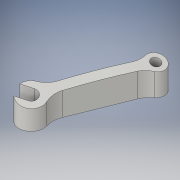
# Autodesk Inventor part: Team Pin Mechanical-Left Wrench
Saved by Autodesk Inventor 2016 (Build 200138000, 138)
## iProperties
Created: 2016-02-20
Part Number: Team Pin Mechanical-Left Wrench
Material: Generic
Document SubType Name: Modeling
Designer: RoksBot
Density: 1 g/cm^3
Appearance: White
Author: RoksBot
Autodesk Inventor part; units mm, degrees
ref_plane "YZ Plane" through (0, 0, 0) normal (1, 0, 0) x (0, 1, 0)
ref_plane "XZ Plane" through (0, 0, 0) normal (0, 1, 0) x (-1, 0, 0)
ref_plane "XY Plane" through (0, 0, 0) normal (0, 0, 1) x (1, 0, 0)
sketch "Sketch1" plane through (0, 0, 0) normal (0, 0, 1) x (1, 0, 0)
  line L0 (0, 0) -> (0, 8.6646) construction
  line L1 (20.9931, 1.27) -> (20.9931, 5.715)
  line L2 (20.9931, 5.715) -> (27.9781, 3.81)
  line L3 (27.9781, 3.81) -> (27.9781, 0)
  line L4 (27.9781, 0) -> (20.9931, 0)
  line L5 (20.9931, 1.27) -> (18.4531, 1.27)
  line L6 (18.4531, 1.27) -> (18.4531, 0)
  line L7 (18.4531, 0) -> (20.9931, 0)
  dimension "d0" = 20.9931
  dimension "d1" = 4.445
  dimension "d2" = 1.27
  dimension "d3" = 2.54
  dimension "d4" = 3.81
  dimension "d5" = 6.985
  constraints: 16 end point, 2 parallel, 2 perpendicular, 2 vertical, 1 horizontal, 1 horizontal alignment
  measures "d0" distance between parallel lines of L0 L1
  measures "d1" distance from line of L5 L1.end
  measures "d2" distance of L5.end L6.end
  measures "d3" distance between parallel lines of L1 L6
  measures "d4" distance of L2.end L3.end
  measures "d5" distance between parallel lines of L1 L3
revolve "Revolution1" add sketch "Sketch1" angle 360 about axis through (0, 0, 0) along (0, 1, 0)
ref_plane "Work Plane1" through (0, 3.81, 0) normal (0, 1, 0) x (1, 0, 0)
sketch "Sketch2" plane through (0, 0, 0) normal (0, -1, 0) x (1, 0, 0)
  line L0 (0, 0) -> (-45.8206, 0) construction
  circle A0 centre (0, 0) radius 27.9781 projected
  line L1 (-27.6227, 4.445) -> (-30.5181, 2.54)
  line L2 (-30.5181, 2.54) -> (-30.5181, -2.54)
  line L3 (-30.5181, -2.54) -> (-27.6227, -4.445)
  dimension "d7" = 2.54
  dimension "d8" = 8.89
  dimension "d9" = 5.08
  constraints: 8 end point, 2 point on circle, 1 equal length, 1 horizontal, 1 vertical, 1 other
  measures "d7" distance edge to line of A0 L2
  measures "d8" distance of L3.end L1.start
  measures "d9" distance of L1.end L2.end
extrude "Extrusion1" add sketch "Sketch2" against normal up to surface (3.81 mm away) contours A0 L3 L2 L1
pattern_circular "Circular Pattern1" count 12 over 360 about axis through (0, 1.905, 0) along (0, -1, 0) of "Extrusion1"
sketch "Sketch3" plane through (0, 1.27, 0) normal (0, 1, 0) x (1, 0, 0)
  circle A0 centre (0, 0) radius 18.4531 projected
  circle A1 centre (0, 0) radius 18.4531 projected
  circle A2 centre (0, 0) radius 20.9931 projected
  circle A3 centre (0, 0) radius 20.9931 projected
  arc A4 (-26.1445, 9.9619) -> (-27.6227, 4.445) centre (0, 0) ccw projected
  arc A5 (-27.6227, 4.445) -> (-27.6227, -4.445) centre (0, 0) ccw projected
  arc A6 (-27.6227, -4.445) -> (-26.1445, -9.9619) centre (0, 0) ccw projected
  arc A7 (-26.1445, -9.9619) -> (-21.6995, -17.6609) centre (0, 0) ccw projected
  arc A8 (-21.6995, -17.6609) -> (-17.6609, -21.6995) centre (0, 0) ccw projected
  arc A9 (-17.6609, -21.6995) -> (-9.9619, -26.1445) centre (0, 0) ccw projected
  arc A10 (-9.9619, -26.1445) -> (-4.445, -27.6227) centre (0, 0) ccw projected
  arc A11 (-4.445, -27.6227) -> (4.445, -27.6227) centre (0, 0) ccw projected
  arc A12 (4.445, -27.6227) -> (9.9619, -26.1445) centre (0, 0) ccw projected
  arc A13 (9.9619, -26.1445) -> (17.6609, -21.6995) centre (0, 0) ccw projected
  arc A14 (17.6609, -21.6995) -> (21.6995, -17.6609) centre (0, 0) ccw projected
  arc A15 (21.6995, -17.6609) -> (26.1445, -9.9619) centre (0, 0) ccw projected
  arc A16 (26.1445, -9.9619) -> (27.6227, -4.445) centre (0, 0) ccw projected
  arc A17 (27.6227, -4.445) -> (27.6227, 4.445) centre (0, 0) ccw projected
  arc A18 (27.6227, 4.445) -> (26.1445, 9.9619) centre (0, 0) ccw projected
  arc A19 (26.1445, 9.9619) -> (21.6995, 17.6609) centre (0, 0) ccw projected
  arc A20 (21.6995, 17.6609) -> (17.6609, 21.6995) centre (0, 0) ccw projected
  arc A21 (17.6609, 21.6995) -> (9.9619, 26.1445) centre (0, 0) ccw projected
  arc A22 (9.9619, 26.1445) -> (4.445, 27.6227) centre (0, 0) ccw projected
  arc A23 (4.445, 27.6227) -> (-4.445, 27.6227) centre (0, 0) ccw projected
  arc A24 (-4.445, 27.6227) -> (-9.9619, 26.1445) centre (0, 0) ccw projected
  arc A25 (-9.9619, 26.1445) -> (-17.6609, 21.6995) centre (0, 0) ccw projected
  arc A26 (-17.6609, 21.6995) -> (-21.6995, 17.6609) centre (0, 0) ccw projected
  arc A27 (-21.6995, 17.6609) -> (-26.1445, 9.9619) centre (0, 0) ccw projected
  circle A28 centre (0, 0) radius 22.8981
  spline S0 degree 2 poles (-20.4865, -10.8927) (-20.2314, -10.7347) (-20.0767, -10.9844) knots 0 0 0 1 1 1
  spline S1 degree 2 poles (-20.0767, -10.9844) (-19.9219, -11.2342) (-20.177, -11.3922) knots 0 0 0 1 1 1
  line L0 (-20.177, -11.3922) -> (-22.4984, -12.8306)
  line L1 (-22.4984, -12.8306) -> (-21.0657, -12.8234)
  spline S2 degree 2 poles (-21.0657, -12.8234) (-20.8353, -12.8371) (-20.7343, -13.0001) knots 0 0 0 1 1 1
  spline S3 degree 2 poles (-20.7343, -13.0001) (-20.6366, -13.1578) (-20.7235, -13.3463) knots 0 0 0 1 1 1
  line L2 (-20.7235, -13.3463) -> (-21.4078, -14.6436)
  line L3 (-21.4078, -14.6436) -> (-19.0627, -13.1905)
  spline S4 degree 2 poles (-19.0627, -13.1905) (-18.8077, -13.0325) (-18.6529, -13.2822) knots 0 0 0 1 1 1
  spline S5 degree 2 poles (-18.6529, -13.2822) (-18.4949, -13.5373) (-18.7499, -13.6953) knots 0 0 0 1 1 1
  line L4 (-18.7499, -13.6953) -> (-21.6577, -15.497)
  spline S6 degree 2 poles (-21.6577, -15.497) (-21.9259, -15.6631) (-22.0936, -15.3923) knots 0 0 0 1 1 1
  spline S7 degree 2 poles (-22.0936, -15.3923) (-22.2093, -15.2057) (-22.1246, -15.0076) knots 0 0 0 1 1 1
  line L5 (-22.1246, -15.0076) -> (-21.3965, -13.3994)
  line L6 (-21.3965, -13.3994) -> (-23.1279, -13.3298)
  spline S8 degree 2 poles (-23.1279, -13.3298) (-23.414, -13.3142) (-23.5248, -13.1355) knots 0 0 0 1 1 1
  spline S9 degree 2 poles (-23.5248, -13.1355) (-23.5932, -13.025) (-23.5178, -12.7709) (-23.3942, -12.6944) knots 0 0 0 1 2 2 2
  line L7 (-23.3942, -12.6944) -> (-20.4865, -10.8927)
  line L8 (-21.4115, -8.1592) -> (-20.6563, -9.942)
  line L9 (-20.6563, -9.942) -> (-23.6894, -11.2268)
  line L10 (-23.6894, -11.2268) -> (-24.4445, -9.444)
  spline S10 degree 2 poles (-24.4445, -9.444) (-24.5591, -9.1734) (-24.2914, -9.06) knots 0 0 0 1 1 1
  spline S11 degree 2 poles (-24.2914, -9.06) (-24.0209, -8.9454) (-23.9063, -9.216) knots 0 0 0 1 1 1
  line L11 (-23.9063, -9.216) -> (-23.3743, -10.4719)
  line L12 (-23.3743, -10.4719) -> (-22.8189, -10.2367)
  line L13 (-22.8189, -10.2367) -> (-23.3171, -9.0605)
  spline S12 degree 2 poles (-23.3171, -9.0605) (-23.4293, -8.7956) (-23.1616, -8.6822) knots 0 0 0 1 1 1
  spline S13 degree 2 poles (-23.1616, -8.6822) (-22.8854, -8.5652) (-22.7732, -8.8301) knots 0 0 0 1 1 1
  line L14 (-22.7732, -8.8301) -> (-22.275, -10.0063)
  line L15 (-22.275, -10.0063) -> (-21.4235, -9.6456)
  line L16 (-21.4235, -9.6456) -> (-21.9554, -8.3897)
  spline S14 degree 2 poles (-21.9554, -8.3897) (-22.07, -8.1191) (-21.8023, -8.0057) knots 0 0 0 1 1 1
  spline S15 degree 2 poles (-21.8023, -8.0057) (-21.5261, -7.8887) (-21.4115, -8.1592) knots 0 0 0 1 1 1
  spline S16 degree 2 poles (-22.8056, -5.2377) (-22.4484, -5.3877) (-22.1014, -5.7752) (-22.015, -6.0818) knots 0 0 0 1 2 2 2
  spline S17 degree 2 poles (-22.015, -6.0818) (-21.8732, -6.5849) (-22.313, -7.0655) knots 0 0 0 1 1 1
  spline S18 degree 2 poles (-22.313, -7.0655) (-22.5945, -7.4918) (-23.3387, -7.7016) knots 0 0 0 1 1 1
  spline S19 degree 2 poles (-23.3387, -7.7016) (-24.1544, -7.9314) (-24.69, -7.6614) knots 0 0 0 1 1 1
  spline S20 degree 2 poles (-24.69, -7.6614) (-25.1213, -7.4423) (-25.2479, -6.9928) knots 0 0 0 1 1 1
  spline S21 degree 2 poles (-25.2479, -6.9928) (-25.3444, -6.6505) (-25.2198, -6.1462) (-24.9563, -5.8953) knots 0 0 0 1 2 2 2
  spline S22 degree 2 poles (-24.9563, -5.8953) (-24.9018, -5.8381) (-24.8303, -5.818) knots 0 0 0 1 1 1
  spline S23 degree 2 poles (-24.8303, -5.818) (-24.7112, -5.7844) (-24.4997, -5.908) (-24.4678, -6.0211) knots 0 0 0 1 2 2 2
  spline S24 degree 2 poles (-24.4678, -6.0211) (-24.4242, -6.1759) (-24.5806, -6.3164) knots 0 0 0 1 1 1
  spline S25 degree 2 poles (-24.5806, -6.3164) (-24.7683, -6.517) (-24.6827, -6.8207) knots 0 0 0 1 1 1
  spline S26 degree 2 poles (-24.6827, -6.8207) (-24.6139, -7.0648) (-24.3475, -7.1664) knots 0 0 0 1 1 1
  spline S27 degree 2 poles (-24.3475, -7.1664) (-24.0157, -7.2947) (-23.4948, -7.1479) knots 0 0 0 1 1 1
  spline S28 degree 2 poles (-23.4948, -7.1479) (-23.0095, -7.0111) (-22.5148, -6.4861) (-22.587, -6.2301) knots 0 0 0 1 2 2 2
  spline S29 degree 2 poles (-22.587, -6.2301) (-22.6767, -5.9116) (-22.9983, -5.774) knots 0 0 0 1 1 1
  spline S30 degree 2 poles (-22.9983, -5.774) (-23.1807, -5.7194) (-23.2168, -5.5914) knots 0 0 0 1 1 1
  spline S31 degree 2 poles (-23.2168, -5.5914) (-23.2487, -5.4783) (-23.1196, -5.2523) (-23.0064, -5.2204) knots 0 0 0 1 2 2 2
  spline S32 degree 2 poles (-23.0064, -5.2204) (-22.9082, -5.1928) (-22.8056, -5.2377) knots 0 0 0 1 1 1
  spline S33 degree 2 poles (-23.0841, -2.194) (-22.7873, -2.1504) (-22.7455, -2.435) knots 0 0 0 1 1 1
  spline S34 degree 2 poles (-22.7455, -2.435) (-22.7028, -2.7257) (-22.9996, -2.7693) knots 0 0 0 1 1 1
  line L17 (-22.9996, -2.7693) -> (-24.1563, -2.9392)
  line L18 (-24.1563, -2.9392) -> (-23.9877, -4.0867)
  line L19 (-23.9877, -4.0867) -> (-22.8311, -3.9168)
  spline S35 degree 2 poles (-22.8311, -3.9168) (-22.5342, -3.8732) (-22.4915, -4.1639) knots 0 0 0 1 1 1
  spline S36 degree 2 poles (-22.4915, -4.1639) (-22.4488, -4.4546) (-22.7456, -4.4982) knots 0 0 0 1 1 1
  line L20 (-22.7456, -4.4982) -> (-25.4599, -4.8969)
  spline S37 degree 2 poles (-25.4599, -4.8969) (-25.7536, -4.9401) (-25.7963, -4.6494) knots 0 0 0 1 1 1
  spline S38 degree 2 poles (-25.7963, -4.6494) (-25.839, -4.3587) (-25.5453, -4.3155) knots 0 0 0 1 1 1
  line L21 (-25.5453, -4.3155) -> (-24.5722, -4.1726)
  line L22 (-24.5722, -4.1726) -> (-24.7408, -3.0251)
  line L23 (-24.7408, -3.0251) -> (-25.7139, -3.168)
  spline S39 degree 2 poles (-25.7139, -3.168) (-26.0076, -3.2112) (-26.0503, -2.9205) knots 0 0 0 1 1 1
  spline S40 degree 2 poles (-26.0503, -2.9205) (-26.0921, -2.6359) (-25.7984, -2.5928) knots 0 0 0 1 1 1
  line L24 (-25.7984, -2.5928) -> (-23.0841, -2.194)
  spline S41 degree 2 poles (-23.2836, 1.208) (-23.2064, 1.2364) (-23.1539, 1.2367) knots 0 0 0 1 1 1
  spline S42 degree 2 poles (-23.1539, 1.2367) (-23.0302, 1.2375) (-22.8651, 1.053) (-22.8643, 0.9323) knots 0 0 0 1 2 2 2
  spline S43 degree 2 poles (-22.8643, 0.9323) (-22.8631, 0.7437) (-23.042, 0.6683) knots 0 0 0 1 1 1
  line L25 (-23.042, 0.6683) -> (-23.4523, 0.5049)
  line L26 (-23.4523, 0.5049) -> (-23.4439, -0.8127)
  line L27 (-23.4439, -0.8127) -> (-23.0192, -0.9677)
  spline S44 degree 2 poles (-23.0192, -0.9677) (-22.8518, -1.0347) (-22.8505, -1.2295) knots 0 0 0 1 1 1
  spline S45 degree 2 poles (-22.8505, -1.2295) (-22.8498, -1.3439) (-23.0064, -1.5305) (-23.1301, -1.5313) knots 0 0 0 1 2 2 2
  spline S46 degree 2 poles (-23.1301, -1.5313) (-23.1826, -1.5316) (-23.2322, -1.5134) knots 0 0 0 1 1 1
  line L28 (-23.2322, -1.5134) -> (-26.0565, -0.4767)
  spline S47 degree 2 poles (-26.0565, -0.4767) (-26.2212, -0.3571) (-26.2222, -0.1963) knots 0 0 0 1 1 1
  spline S48 degree 2 poles (-26.2222, -0.1963) (-26.2233, -0.0262) (-26.0632, 0.0924) knots 0 0 0 1 1 1
  line L29 (-26.0632, 0.0924) -> (-23.2836, 1.208)
  line L30 (-24.0233, 0.3126) -> (-25.2852, -0.1749)
  line L31 (-25.2852, -0.1749) -> (-24.0173, -0.6307)
  line L32 (-24.0173, -0.6307) -> (-24.0233, 0.3126)
  spline S49 degree 2 poles (-22.7917, 4.2665) (-22.4883, 4.2255) (-22.5223, 3.9742) knots 0 0 0 1 1 1
  spline S50 degree 2 poles (-22.5223, 3.9742) (-22.5451, 3.8056) (-22.7963, 3.7022) knots 0 0 0 1 1 1
  line L33 (-22.7963, 3.7022) -> (-24.9996, 2.6644)
  line L34 (-24.9996, 2.6644) -> (-23.038, 2.3991)
  spline S51 degree 2 poles (-23.038, 2.3991) (-22.7407, 2.3589) (-22.7793, 2.0739) knots 0 0 0 1 1 1
  spline S52 degree 2 poles (-22.7793, 2.0739) (-22.8178, 1.7888) (-23.1151, 1.8291) knots 0 0 0 1 1 1
  line L35 (-23.1151, 1.8291) -> (-25.8582, 2.2)
  spline S53 degree 2 poles (-25.8582, 2.2) (-26.1463, 2.239) (-26.109, 2.5148) knots 0 0 0 1 1 1
  spline S54 degree 2 poles (-26.109, 2.5148) (-26.0867, 2.6803) (-25.9475, 2.6709) knots 0 0 0 1 1 1
  line L36 (-25.9475, 2.6709) -> (-23.6718, 3.805)
  line L37 (-23.6718, 3.805) -> (-25.5813, 4.0632)
  spline S55 degree 2 poles (-25.5813, 4.0632) (-25.8755, 4.103) (-25.837, 4.3881) knots 0 0 0 1 1 1
  spline S56 degree 2 poles (-25.837, 4.3881) (-25.7984, 4.6731) (-25.5042, 4.6333) knots 0 0 0 1 1 1
  line L38 (-25.5042, 4.6333) -> (-22.7917, 4.2665)
  spline S57 degree 2 poles (-22.4654, 5.6266) (-22.1736, 5.5569) (-22.2419, 5.2711) knots 0 0 0 1 1 1
  spline S58 degree 2 poles (-22.2419, 5.2711) (-22.3101, 4.9853) (-22.6019, 5.055) knots 0 0 0 1 1 1
  line L39 (-22.6019, 5.055) -> (-25.2702, 5.6925)
  spline S59 degree 2 poles (-25.2702, 5.6925) (-25.559, 5.7615) (-25.4907, 6.0473) knots 0 0 0 1 1 1
  spline S60 degree 2 poles (-25.4907, 6.0473) (-25.4224, 6.3331) (-25.1336, 6.2641) knots 0 0 0 1 1 1
  line L40 (-25.1336, 6.2641) -> (-22.4654, 5.6266)
  spline S61 degree 2 poles (-21.7348, 8.6674) (-21.5264, 8.3409) (-21.4615, 7.8248) (-21.5649, 7.5235) knots 0 0 0 1 2 2 2
  spline S62 degree 2 poles (-21.5649, 7.5235) (-21.7346, 7.0291) (-22.3696, 6.8841) knots 0 0 0 1 1 1
  spline S63 degree 2 poles (-22.3696, 6.8841) (-22.8437, 6.6936) (-23.5751, 6.9445) knots 0 0 0 1 1 1
  spline S64 degree 2 poles (-23.5751, 6.9445) (-24.3766, 7.2196) (-24.6635, 7.7463) knots 0 0 0 1 1 1
  spline S65 degree 2 poles (-24.6635, 7.7463) (-24.8935, 8.1719) (-24.7419, 8.6136) knots 0 0 0 1 1 1
  spline S66 degree 2 poles (-24.7419, 8.6136) (-24.6265, 8.95) (-24.2371, 9.2938) (-23.8777, 9.3503) knots 0 0 0 1 2 2 2
  spline S67 degree 2 poles (-23.8777, 9.3503) (-23.8003, 9.3663) (-23.7301, 9.3422) knots 0 0 0 1 1 1
  spline S68 degree 2 poles (-23.7301, 9.3422) (-23.6131, 9.3021) (-23.5094, 9.0801) (-23.5475, 8.9689) knots 0 0 0 1 2 2 2
  spline S69 degree 2 poles (-23.5475, 8.9689) (-23.5997, 8.8168) (-23.8083, 8.7903) knots 0 0 0 1 1 1
  spline S70 degree 2 poles (-23.8083, 8.7903) (-24.0768, 8.732) (-24.1792, 8.4336) knots 0 0 0 1 1 1
  spline S71 degree 2 poles (-24.1792, 8.4336) (-24.2615, 8.1937) (-24.1002, 7.9585) knots 0 0 0 1 1 1
  spline S72 degree 2 poles (-24.1002, 7.9585) (-23.9003, 7.6643) (-23.3884, 7.4887) knots 0 0 0 1 1 1
  spline S73 degree 2 poles (-23.3884, 7.4887) (-22.9115, 7.3251) (-22.206, 7.4754) (-22.1197, 7.7269) knots 0 0 0 1 2 2 2
  spline S74 degree 2 poles (-22.1197, 7.7269) (-22.0123, 8.04) (-22.1984, 8.336) knots 0 0 0 1 1 1
  spline S75 degree 2 poles (-22.1984, 8.336) (-22.3174, 8.4847) (-22.2743, 8.6105) knots 0 0 0 1 1 1
  spline S76 degree 2 poles (-22.2743, 8.6105) (-22.2361, 8.7217) (-22.0014, 8.8341) (-21.8902, 8.7959) knots 0 0 0 1 2 2 2
  spline S77 degree 2 poles (-21.8902, 8.7959) (-21.7937, 8.7628) (-21.7348, 8.6674) knots 0 0 0 1 1 1
  spline S78 degree 2 poles (-20.1702, 11.694) (-20.0886, 11.684) (-20.0417, 11.6603) knots 0 0 0 1 1 1
  spline S79 degree 2 poles (-20.0417, 11.6603) (-19.9312, 11.6046) (-19.8684, 11.3651) (-19.9228, 11.2574) knots 0 0 0 1 2 2 2
  spline S80 degree 2 poles (-19.9228, 11.2574) (-20.0077, 11.0889) (-20.2013, 11.1035) knots 0 0 0 1 1 1
  line L41 (-20.2013, 11.1035) -> (-20.641, 11.1451)
  line L42 (-20.641, 11.1451) -> (-21.2344, 9.9688)
  line L43 (-21.2344, 9.9688) -> (-20.9272, 9.6371)
  spline S81 degree 2 poles (-20.9272, 9.6371) (-20.8087, 9.5011) (-20.8965, 9.3272) knots 0 0 0 1 1 1
  spline S82 degree 2 poles (-20.8965, 9.3272) (-20.948, 9.225) (-21.1724, 9.1304) (-21.2829, 9.1861) knots 0 0 0 1 2 2 2
  spline S83 degree 2 poles (-21.2829, 9.1861) (-21.3298, 9.2098) (-21.3656, 9.2486) knots 0 0 0 1 1 1
  line L44 (-21.3656, 9.2486) -> (-23.4063, 11.4593)
  spline S84 degree 2 poles (-23.4063, 11.4593) (-23.4983, 11.6408) (-23.4258, 11.7844) knots 0 0 0 1 1 1
  spline S85 degree 2 poles (-23.4258, 11.7844) (-23.3492, 11.9363) (-23.1527, 11.9688) knots 0 0 0 1 1 1
  line L45 (-23.1527, 11.9688) -> (-20.1702, 11.694)
  line L46 (-21.2369, 11.2344) -> (-22.5822, 11.3761)
  line L47 (-22.5822, 11.3761) -> (-21.6617, 10.3922)
  line L48 (-21.6617, 10.3922) -> (-21.2369, 11.2344)
  line L49 (-18.3775, 13.6927) -> (-19.469, 12.0936)
  line L50 (-19.469, 12.0936) -> (-21.9443, 13.7831)
  spline S86 degree 2 poles (-21.9443, 13.7831) (-22.1896, 13.9505) (-22.0274, 14.188) knots 0 0 0 1 1 1
  spline S87 degree 2 poles (-22.0274, 14.188) (-21.867, 14.4231) (-21.6218, 14.2557) knots 0 0 0 1 1 1
  line L51 (-21.6218, 14.2557) -> (-19.6343, 12.8992)
  line L52 (-19.6343, 12.8992) -> (-18.8654, 14.0258)
  spline S88 degree 2 poles (-18.8654, 14.0258) (-18.6998, 14.2684) (-18.4597, 14.1045) knots 0 0 0 1 1 1
  spline S89 degree 2 poles (-18.4597, 14.1045) (-18.2119, 13.9354) (-18.3775, 13.6927) knots 0 0 0 1 1 1
  dimension "d16" = 1.905
  constraints: 1 centre point, 1 coincident, 1 other
  measures "d16" radial gap between concentric circles of A2 A28
extrude "Extrusion2" cut sketch "Sketch3" along normal blind 25.4 contours S5 L4 S6 S7 L5 L6 S8 S9 L7 S0 A28 S1 L0 L1 S2 S3 L2 L3 S4 | L8 L9 L10 S10 S11 L11 L12 L13 S12 S13 L14 L15 L16 S14 S15 | L49 L50 S86 S87 L51 L52 S88 S89 | A28 S0 S1 | S79 S80 A28 | A28 S80 L41 L42 L43 S81 S82 S83 L44 S84 S85 L45 S78 S79 | S17 S18 S19 S20 S21 S22 S23 S24 S25 S26 S27 S28 S29 S30 S31 S32 S16 A28 | A28 S16 S17 | S81 S82 A28 | S36 L20 S37 S38 L21 L22 L23 S39 S40 L24 S33 A28 S34 L17 L18 L19 S35 | A28 S35 S36 | S61 S62 A28 | A28 S62 S63 S64 S65 S66 S67 S68 S69 S70 S71 S72 S73 S74 S75 S76 S77 S61 | A28 S33 S34 | S57 S58 A28 | A28 S58 L39 S59 S60 L40 S57 | S45 S46 L28 S47 S48 L29 S41 S42 A28 S43 L25 L26 L27 S44 | A28 S44 S45 | S49 S50 A28 | A28 S50 L33 L34 S51 S52 L35 S53 S54 L36 L37 S55 S56 L38 S49 | A28 S42 S43 | S51 S52 A28
sketch "Sketch4" plane through (0, 1.27, 0) normal (0, 1, 0) x (1, 0, 0)
  line L0 (-22.7963, 3.7022) -> (-24.9996, 2.6644) projected
  line L1 (-24.9996, 2.6644) -> (-23.038, 2.3991) projected
  line L2 (-23.1151, 1.8291) -> (-25.8582, 2.2) projected
  line L3 (-25.9475, 2.6709) -> (-23.6718, 3.805) projected
  line L4 (-23.6718, 3.805) -> (-25.5813, 4.0632) projected
  line L5 (-25.5042, 4.6333) -> (-22.7917, 4.2665) projected
  line L6 (-23.042, 0.6683) -> (-23.4523, 0.5049) projected
  line L7 (-23.4523, 0.5049) -> (-23.4439, -0.8127) projected
  line L8 (-23.4439, -0.8127) -> (-23.0192, -0.9677) projected
  line L9 (-23.2322, -1.5134) -> (-26.0565, -0.4767) projected
  line L10 (-26.0632, 0.0924) -> (-23.2836, 1.208) projected
  line L11 (-20.177, -11.3922) -> (-22.4984, -12.8306) projected
  line L12 (-22.4984, -12.8306) -> (-21.0657, -12.8234) projected
  line L13 (-20.7235, -13.3463) -> (-21.4078, -14.6436) projected
  line L14 (-21.4078, -14.6436) -> (-19.0627, -13.1905) projected
  line L15 (-18.7499, -13.6953) -> (-21.6577, -15.497) projected
  line L16 (-22.1246, -15.0076) -> (-21.3965, -13.3994) projected
  line L17 (-21.3965, -13.3994) -> (-23.1279, -13.3298) projected
  line L18 (-23.3942, -12.6944) -> (-20.4865, -10.8927) projected
  line L19 (-20.6563, -9.942) -> (-23.6894, -11.2268) projected
  line L20 (-23.6894, -11.2268) -> (-24.4445, -9.444) projected
  line L21 (-23.9063, -9.216) -> (-23.3743, -10.4719) projected
  line L22 (-23.3743, -10.4719) -> (-22.8189, -10.2367) projected
  line L23 (-22.8189, -10.2367) -> (-23.3171, -9.0605) projected
  line L24 (-22.7732, -8.8301) -> (-22.275, -10.0063) projected
  line L25 (-22.275, -10.0063) -> (-21.4235, -9.6456) projected
  line L26 (-21.4235, -9.6456) -> (-21.9554, -8.3897) projected
  line L27 (-21.4115, -8.1592) -> (-20.6563, -9.942) projected
  line L28 (-22.9996, -2.7693) -> (-24.1563, -2.9392) projected
  line L29 (-24.1563, -2.9392) -> (-23.9877, -4.0867) projected
  line L30 (-23.9877, -4.0867) -> (-22.8311, -3.9168) projected
  line L31 (-22.7456, -4.4982) -> (-25.4599, -4.8969) projected
  line L32 (-25.5453, -4.3155) -> (-24.5722, -4.1726) projected
  line L33 (-24.5722, -4.1726) -> (-24.7408, -3.0251) projected
  line L34 (-24.7408, -3.0251) -> (-25.7139, -3.168) projected
  line L35 (-25.7984, -2.5928) -> (-23.0841, -2.194) projected
  line L36 (-22.6019, 5.055) -> (-25.2702, 5.6925) projected
  line L37 (-25.1336, 6.2641) -> (-22.4654, 5.6266) projected
  line L38 (-20.2013, 11.1035) -> (-20.641, 11.1451) projected
  line L39 (-20.641, 11.1451) -> (-21.2344, 9.9688) projected
  line L40 (-21.2344, 9.9688) -> (-20.9272, 9.6371) projected
  line L41 (-21.3656, 9.2486) -> (-23.4063, 11.4593) projected
  line L42 (-23.1527, 11.9688) -> (-20.1702, 11.694) projected
  line L43 (-19.469, 12.0936) -> (-21.9443, 13.7831) projected
  line L44 (-21.6218, 14.2557) -> (-19.6343, 12.8992) projected
  line L45 (-19.6343, 12.8992) -> (-18.8654, 14.0258) projected
  line L46 (-18.3775, 13.6927) -> (-19.469, 12.0936) projected
  circle A0 centre (0, 0) radius 20.9931 projected
  arc A1 (-26.1445, 9.9619) -> (-27.6227, 4.445) centre (0, 0) ccw projected
  arc A2 (-27.6227, 4.445) -> (-27.6227, -4.445) centre (0, 0) ccw projected
  arc A3 (-27.6227, -4.445) -> (-26.1445, -9.9619) centre (0, 0) ccw projected
  arc A4 (-26.1445, -9.9619) -> (-21.6995, -17.6609) centre (0, 0) ccw projected
  arc A5 (-21.6995, -17.6609) -> (-17.6609, -21.6995) centre (0, 0) ccw projected
  arc A6 (-17.6609, -21.6995) -> (-9.9619, -26.1445) centre (0, 0) ccw projected
  arc A7 (-9.9619, -26.1445) -> (-4.445, -27.6227) centre (0, 0) ccw projected
  arc A8 (-4.445, -27.6227) -> (4.445, -27.6227) centre (0, 0) ccw projected
  arc A9 (4.445, -27.6227) -> (9.9619, -26.1445) centre (0, 0) ccw projected
  arc A10 (9.9619, -26.1445) -> (17.6609, -21.6995) centre (0, 0) ccw projected
  arc A11 (17.6609, -21.6995) -> (21.6995, -17.6609) centre (0, 0) ccw projected
  arc A12 (21.6995, -17.6609) -> (26.1445, -9.9619) centre (0, 0) ccw projected
  arc A13 (26.1445, -9.9619) -> (27.6227, -4.445) centre (0, 0) ccw projected
  arc A14 (27.6227, -4.445) -> (27.6227, 4.445) centre (0, 0) ccw projected
  arc A15 (27.6227, 4.445) -> (26.1445, 9.9619) centre (0, 0) ccw projected
  arc A16 (26.1445, 9.9619) -> (21.6995, 17.6609) centre (0, 0) ccw projected
  arc A17 (21.6995, 17.6609) -> (17.6609, 21.6995) centre (0, 0) ccw projected
  arc A18 (17.6609, 21.6995) -> (9.9619, 26.1445) centre (0, 0) ccw projected
  arc A19 (9.9619, 26.1445) -> (4.445, 27.6227) centre (0, 0) ccw projected
  arc A20 (4.445, 27.6227) -> (-4.445, 27.6227) centre (0, 0) ccw projected
  arc A21 (-4.445, 27.6227) -> (-9.9619, 26.1445) centre (0, 0) ccw projected
  arc A22 (-9.9619, 26.1445) -> (-17.6609, 21.6995) centre (0, 0) ccw projected
  arc A23 (-17.6609, 21.6995) -> (-21.6995, 17.6609) centre (0, 0) ccw projected
  arc A24 (-21.6995, 17.6609) -> (-26.1445, 9.9619) centre (0, 0) ccw projected
  circle A25 centre (0, 0) radius 18.4531 projected
  circle A26 centre (0, 0) radius 20.9931 projected
  circle A27 centre (24.1681, -3.81) radius 1.27
  circle A28 centre (24.1681, -3.81) radius 0.635
  line L47 (30.5181, 2.54) -> (30.5181, -2.54) projected
  arc A29 (17.9659, -17.8891) -> (17.3155, -16.3716) centre (19.0881, -16.51) ccw
  line L48 (19.0881, -16.51) -> (15.2571, -18.1519) construction
  line L49 (18.7629, -15.7512) -> (17.3155, -16.3716)
  line L50 (17.9659, -17.8891) -> (19.4133, -17.2688)
  arc A30 (19.4133, -17.2688) -> (18.7629, -15.7512) centre (19.0881, -16.51) ccw
  line L51 (19.0881, -16.51) -> (24.1681, -3.81) construction
  line L52 (19.1153, -14.7322) -> (23.17, -4.5954)
  line L53 (20.2945, -15.2039) -> (24.3492, -5.067)
  line L54 (0, 0) -> (36.9495, 0) construction
  arc A31 (26.1445, 9.9619) -> (21.6995, 17.6609) centre (0, 0) ccw
  arc A32 (27.6227, 4.445) -> (26.1445, 9.9619) centre (0, 0) ccw
  circle A33 centre (24.1681, 3.81) radius 1.27
  circle A34 centre (24.1681, 3.81) radius 0.635
  arc A35 (17.3155, 16.3716) -> (17.9659, 17.8891) centre (19.0881, 16.51) ccw
  line L55 (19.0881, 16.51) -> (15.2571, 18.1519) construction
  line L56 (18.7629, 15.7512) -> (17.3155, 16.3716)
  line L57 (17.9659, 17.8891) -> (19.4133, 17.2688)
  arc A36 (18.7629, 15.7512) -> (19.4133, 17.2688) centre (19.0881, 16.51) ccw
  line L58 (19.0881, 16.51) -> (24.1681, 3.81) construction
  line L59 (19.1153, 14.7322) -> (23.17, 4.5954)
  line L60 (20.2945, 15.2039) -> (24.3492, 5.067)
  point P0 (17.1726, -17.3309)
  point P1 (17.1726, 17.3309)
  dimension "d19" = 2.54
  dimension "d20" = 0.635
  dimension "d22" = 3.81
  dimension "d23" = 6.35
  dimension "d24" = 3.556
  dimension "d25" = 135
  dimension "d26" = 1.27
  dimension "d27" = 0.635
  dimension "d28" = 12.7
  dimension "d29" = 5.08
  dimension "d30" = 1.651
  constraints: 30 end point, 20 point on circle, 13 symmetric about line, 10 centre point, 4 parallel, 2 coincident, 2 tangent, 1 horizontal, 1 midpoint, 96 other
  measures "d19" diameter of A27
  measures "d20" radial gap between concentric circles of A27 A28
  measures "d22" vertical distance of L54.start L51.end
  measures "d23" distance from line of L47 L51.end
  measures "d24" diameter of A29
  measures "d25" angle of L48 L51
  measures "d26" distance between parallel lines of L53 L52
  measures "d27" distance between parallel lines of L52 L51
  measures "d28" vertical distance of L48.start L51.end
  measures "d29" horizontal distance of A27.centre L48.start
  measures "d30" distance between parallel lines of L50 L49
extrude "Extrusion3" cut sketch "Sketch4" along normal through all contours A27 | A27 L53 A29 L52 | A29 L50 A30 L49 keep common part
fillet "Fillet1" radius 3.175 4 edges at (19.1153, 3.0642, 14.7322) (20.2945, 2.8973, 15.2039) (23.17, 3.1341, 4.5954) (24.3492, 2.9637, 5.067)
equation "\"d27\" = 0.5 * d26"
body "Solid1"
